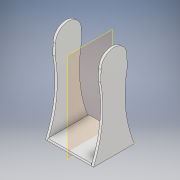
# Autodesk Inventor part: MAN_BASIS_PRIMARY_STRUCTURE
Saved by Autodesk Inventor 2019 (Build 230136000, 136)
## iProperties
Created: 2021-03-07
Part Number: MAN_BASIS_PRIMARY_STRUCTURE
Material: ABS Plastic
Document SubType Name: Modeling
Designer: DOMEK
Density: 1.06 g/cm^3
Appearance: Smooth - White
Author: DOMEK
Autodesk Inventor part; units mm, degrees
ref_plane "YZ Plane" through (0, 0, 0) normal (1, 0, 0) x (0, 1, 0)
ref_plane "XZ Plane" through (0, 0, 0) normal (0, 1, 0) x (-1, 0, 0)
ref_plane "XY Plane" through (0, 0, 0) normal (0, 0, 1) x (1, 0, 0)
sketch "Sketch7" plane through (0, 0, 0) normal (0, 1, 0) x (-1, 0, 0)
  line L0 (0, 0) -> (41, 0)
  line L1 (41, 0) -> (41, 35)
  line L2 (41, 35) -> (0, 35)
  line L3 (0, 35) -> (0, 0)
  dimension "d20" = 41
  dimension "d21" = 35
  constraints: 8 end point, 2 parallel, 1 horizontal, 1 perpendicular
  measures "d20" distance of L2.end L1.end
  measures "d21" distance of L1.end L0.end
extrude "Extrusion6" add sketch "Sketch7" along normal blind 80
shell "Shell1" thickness 2 removed faces 3 at (-13.6667, 80, 23.3333) at (-27.3333, 26.6667, 35) at (-13.6667, 26.6667, 0)
sketch "Sketch8" plane through (0, 0, 35) normal (1, 0, 0) x (0, 0, -1)
  point P0 (35, 0)
sketch "Sketch9" plane through (0, 0, 35) normal (1, 0, 0) x (0, 0, -1)
  line L0 (0, 80) -> (35, 80) projected
  line L1 (17.5, 80) -> (17.5, 0)
  arc A0 (35, 80) -> (35, 0) centre (130.4732, 40) ccw
  arc A1 (0, 0) -> (0, 80) centre (-95.4732, 40) ccw
  line L2 (35, 80) -> (35, 2) projected
  line L3 (35, 0) -> (35, 80)
  line L4 (35, 0) -> (0, 0) projected
  line L5 (0, 0) -> (0, 80) projected
  line L6 (0, 0) -> (0, 80)
  constraints: 6 end point, 4 point on circle, 2 centre point, 2 collinear, 2 symmetric about line, 1 midpoint, 1 vertical, 1 other
extrude "Extrusion7" cut sketch "Sketch9" against normal blind 2 contours A1 L5 | L2 L3 A0
ref_plane "Work Plane6" through (-20.5, 0, 35) normal (1, 0, 0) x (0, 0, -1)
mirror "Mirror3" about plane through (-20.5, 0, 35) normal (1, 0, 0) of "Extrusion7"
sketch "Sketch11" plane through (0, 0, 35) normal (1, 0, 0) x (0, 0, -1)
  line L0 (0, 80) -> (35, 80) projected
  circle A0 centre (17.5, 69) radius 11
  arc A1 (35, 80) -> (35, 0) centre (130.4732, 40) ccw projected
  arc A2 (0, 0) -> (0, 80) centre (-95.4732, 40) ccw projected
  line L1 (28.5, 69) -> (28.845, 59.6685)
  line L2 (6.5, 69) -> (6.155, 59.6685)
  dimension "d35" = 22
  constraints: 4 end point, 4 point on circle, 1 centre point
  measures "d35" diameter of A0
extrude "Extrusion9" cut sketch "Sketch11" against normal blind 2 contours L0 A0 L2 A2 | L0 A1 L1 A0
mirror "Mirror5" about plane through (-20.5, 0, 35) normal (1, 0, 0) of "Extrusion9"
body "Solid2"
